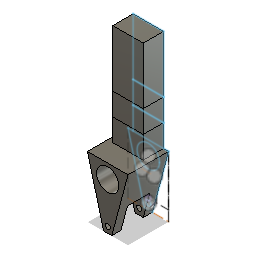
oil-pump-1 (Autodesk Fusion 360 design; units mm, degrees)
Autodesk Fusion 360 part; units mm, degrees
sketch "Sketch1" plane through (0, 0, 0) normal (0, 0, 1) x (1, 0, 0) in component "Component"
  line L0 (0, 0) -> (1, 0) construction
  line L1 (1, 0) -> (1, 2.5) construction
  line L2 (-1, 2.5) -> (-1, -0.5) construction
  line L3 (-1, -0.5) -> (1, -0.5) construction
  line L4 (1, -0.5) -> (1, 2.5) construction
  circle A0 centre (0, -0.2) radius 0.125
  line L5 (-1, 2.5) -> (-0.2008, -0.5)
  line L6 (-0.2008, -0.5) -> (0.2, -0.5)
  line L7 (0.2, -0.5) -> (1, 2.5)
  line L8 (-1, 2.5) -> (1, 2.5)
  line L9 (-0.3, 1.1) -> (0.3, 1.1) construction
  line L10 (-0.75, 2.5) -> (-0.75, 3.6)
  line L11 (-0.75, 3.6) -> (0.75, 3.6)
  line L12 (0.75, 3.6) -> (0.75, 2.5)
  line L13 (-0.75, 3.6) -> (0.75, 3.6)
  line L14 (0.75, 3.6) -> (0.75, 4.7)
  line L15 (0.75, 4.7) -> (-0.75, 4.7)
  line L16 (-0.75, 4.7) -> (-0.75, 3.6)
  line L17 (0.75, 4.7) -> (-0.75, 4.7)
  line L18 (-0.75, 4.7) -> (-0.75, 7.5)
  line L19 (-0.75, 7.5) -> (0.75, 7.5)
  line L20 (0.75, 7.5) -> (0.75, 4.7)
  circle A1 centre (0, 1.8) radius 0.55
  dimension "d1" = 1
  dimension "d3" = 2
  dimension "d4" = 3
  dimension "d5" = 0.25
  dimension "d19" = 1.1
  constraint horizontal L0
  constraint vertical L1
  constraint coincident L0.start origin
  constraint vertical L2
  constraint horizontal L3
  constraint vertical L4
  constraint coincident L3 L5.end
  constraint coincident L3 L6.end
  constraint perpendicular L4 L8
  constraint vertical L10
  constraint horizontal L11
  constraint vertical L12
  constraint horizontal L13
  constraint vertical L14
  constraint horizontal L15
  constraint vertical L16
  constraint coincident L8 L12.end
  constraint coincident L8 L10.start
  constraint horizontal L17
  constraint vertical L18
  constraint horizontal L19
  constraint vertical L20
  measures "d1" distance of L0.start L0.end
  measures "d3" distance of L1.end L2.start
  measures "d4" distance of L1.end L3.end
  measures "d5" diameter of A0
  measures "d19" diameter of A1
extrude "Extrude1" add sketch "Sketch1" along normal blind 2 contours L5 L6 L7 L8 makes body 1 in component "Component"
extrude "Extrude2" add sketch "Sketch1" along normal blind 1 contours L8 L10 L11 L12 L13 bodies 1 in component "Component"
extrude "Extrude3" add sketch "Sketch1" along normal blind 1 separate body contours L11 L13 L14 L15 L16 L17 makes body 2 in component "Component"
extrude "Extrude4" add sketch "Sketch1" along normal blind 1 separate body contours L15 L17 L18 L19 L20 makes body 3 in component "Component"
sketch "Sketch2" plane through (0, -0.5, 0) normal (0, -1, 0) x (1, 0, 0) in component "Component"
  line L0 (-0.2008, 0) -> (0.2, 0)
  line L1 (0.2, 0) -> (0.2, 2)
  line L2 (0.2, 2) -> (-0.2008, 2)
  line L3 (-0.2008, 2) -> (-0.2008, 0)
  line L4 (1.4, 1.55) -> (-1.4, 1.55)
  line L5 (-1.4, 1.55) -> (-1.4, 0.45)
  line L6 (-1.4, 0.45) -> (1.4, 0.45)
  line L7 (1.4, 0.45) -> (1.4, 1.55)
  line L8 (1.4, 1.55) -> (-1.4, 0.45) construction
  line L9 (-1.4, 1.55) -> (1.4, 0.45) construction
  point P0 (0, 1)
  dimension "d16" = 1.1
  constraint horizontal L4
  constraint perpendicular L4 L5
  constraint parallel L4 L6
  constraint parallel L5 L7
  constraint coincident L8 P0
  constraint coincident L9 P0
  measures "d16" distance of L4.end L5.end
extrude "Extrude5" cut sketch "Sketch2" against normal blind 1.2 contours L3 L4 L5 L6 | L1 L3 L4 L6 | L1 L4 L6 L7 bodies 1 in component "Component"
component "Component" placed x (1, 0, 0) y (0, 1, 0) z (0, 0, 1) at (0, 0, 0)
